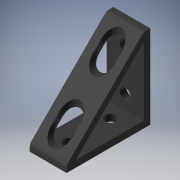
# Autodesk Inventor part: 25-4136 Aluminum
Saved by Autodesk Inventor 2025 (Build 290162000, 162)
## iProperties
Created: 2024-04-27
Part Number: 25-4136 Aluminum
Material: Generic
Catalog Web Link: www.cadenas.de
Description: 25-4136, 40-4336, 30-4366, 45-4366, 25-4136-Black, 40-4336-Black, 30-4366-Black, 45-4366-Black-4 Hole Inside Gusset Corner Bracket
Vendor: 8020
Document SubType Name: Modeling
Designer: psAdmin
Manufacturer: 8020
Mass: 11.5533 g
Surface Area: 77.0782 cm^2
Volume: 11.5533 cm^3
Density: 1 g/cm^3
Appearance: PSOLRGB-191-191-191
Category: PARTsolutions
Company: 8020
PSOL_IDENT_0: {$CADENAS_DATA/23d-libs/8020/metric/joining_plates/25_4136.prj},242 {VTYP=3D},{NB=25-4136},{LINA=25-
PSOL_IDENT_1: 4136},{NN=25-4136, 40-4336, 30-4366, 45-4366, 25-4136-Black, 40-4336-Black, 30-4366-Black, 45-4366-B
PSOL_IDENT_2: lack},{DATE=09.11.2023 07:10:07},{GEOMDATE=11.01.2019 21:53:00},{VERSION=},{LINEID=10},{WBVAR=},{WBN
PSOL_IDENT_3: UMERIC=}  {NB=25-4136},{LINA=25-4136},{KT=DUMMY},{PN=25-4136},{SERIES=25},{MATERIAL=Aluminum},{GRADE=
PSOL_IDENT_4: 6105-T5},{FINISH=Clear Anodize},{A=22.00},{B=50.00},{C=50.00},{D=12.50},{E=12.50},{F=6.81},{G=25.00}
PSOL_IDENT_5: ,{T=4.00},{W=.041},{C1=37.500},{C2=12.500},{C3=12.700},{D1=4.000},{COLOR=.75,.75,.75}
NB: 25-4136
NN: 25-4136, 40-4336, 30-4366, 45-4366, 25-4136-Black, 40-4336-Black, 30-4366-Black, 45-4366-Black
NT: 4 Hole Inside Gusset Corner Bracket
NBSYN: $PN.
LINA: 25-4136
CATALOG: 80/20
PN: 25-4136
SERIES: 25
MATERIAL: Aluminum
GRADE: 6105-T5
FINISH: Clear Anodize
A: 22
B: 50
C: 50
D: 12.5
E: 12.5
F: 6.81
G: 25
T: 4
W: .041
SUPPLIER: 8020
ARTICLENO: 25-4136
BOMINFO: 25-4136
CREATOR: CADENAS GmbH
Title: 25-4136
Author: Cadenas PARTsolutions
Comments: 4 Hole Inside Gusset Corner Bracket
Autodesk Inventor part; units mm, degrees
ref_plane "YZ Plane" through (0, 0, 0) normal (1, 0, 0) x (0, 1, 0)
ref_plane "XZ Plane" through (0, 0, 0) normal (0, 1, 0) x (-1, 0, 0)
ref_plane "XY Plane" through (0, 0, 0) normal (0, 0, 1) x (1, 0, 0)
sketch "Sketch_1" plane through (0, 0, 0) normal (1, 0, 0) x (0, 1, 0)
  line L0 (2.3431, 50) -> (0, 50)
  line L1 (0, 50) -> (0, 0)
  line L2 (0, 0) -> (50, 0)
  line L3 (50, 0) -> (50, 2.3431)
  arc A0 (50, 2.3431) -> (48.8284, 5.1716) centre (46, 2.3431) ccw
  line L4 (48.8284, 5.1716) -> (5.1716, 48.8284)
  arc A1 (5.1716, 48.8284) -> (2.3431, 50) centre (2.3431, 46) ccw
  line L5 (4, 44.3431) -> (4, 4)
  line L6 (4, 4) -> (44.3431, 4)
  line L7 (44.3431, 4) -> (4, 44.3431)
  constraints: 16 end point, 4 point on circle, 2 centre point
extrude "Extrusion1" add sketch "Sketch_1" along normal mid plane 22
sketch "Sketch2" plane through (-11, 0, 0) normal (0, -1, 0) x (1, 0, 0)
  point P0 (11, 12.5)
hole "Hole1" at (0, 0, 12.5) direction (0, 1, 0) diameter 6.81 depth 4
sketch "Sketch3" plane through (11, 50, 0) normal (0, 0, -1) x (-1, 0, 0)
  point P0 (11, -37.5)
hole "Hole2" at (0, 12.5, 0) direction (0, 0, 1) diameter 6.81 depth 4
sketch "Sketch_4" plane through (0, 0, 50) normal (0, 0, 1) x (1, 0, 0)
  circle A0 centre (0, 12.5) radius 6.35
  constraints: 1 centre point
extrude "Extrusion2" cut sketch "Sketch_4" against normal blind 46
sketch "Sketch_5" plane through (0, 50, 0) normal (0, 1, 0) x (1, 0, 0)
  circle A0 centre (0, -12.5) radius 6.35
  constraints: 1 centre point
extrude "Extrusion3" cut sketch "Sketch_5" against normal blind 46
sketch "Sketch6" plane through (11, 50, 0) normal (0, 0, -1) x (-1, 0, 0)
  point P0 (11, -12.5)
hole "Hole3" at (0, 37.5, 0) direction (0, 0, 1) diameter 6.81 depth 4
sketch "Sketch7" plane through (-11, 0, 0) normal (0, -1, 0) x (1, 0, 0)
  point P0 (11, 37.5)
hole "Hole4" at (0, 0, 37.5) direction (0, 1, 0) diameter 6.81 depth 4
sketch "Sketch_8" plane through (0, 0, 50) normal (0, 0, 1) x (1, 0, 0)
  circle A0 centre (0, 37.5) radius 6.35
  constraints: 1 centre point
extrude "Extrusion4" cut sketch "Sketch_8" against normal blind 46
sketch "Sketch_9" plane through (0, 50, 0) normal (0, 1, 0) x (1, 0, 0)
  circle A0 centre (0, -37.5) radius 6.35
  constraints: 1 centre point
extrude "Extrusion5" cut sketch "Sketch_9" against normal blind 46
body "Solid1"
